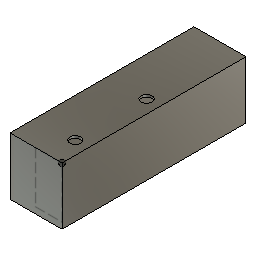
psu-box-115x31x37 (Autodesk Fusion 360 design; units mm, degrees)
Autodesk Fusion 360 part; units mm, degrees
sketch "Sketch1" plane through (0, 0, 0) normal (0, 0, 1) x (1, 0, 0)
  line L0 (0, 0) -> (33.5, 0)
  line L1 (33.5, 0) -> (33.5, 118.5)
  line L2 (33.5, 118.5) -> (0, 118.5)
  line L3 (0, 118.5) -> (0, 0)
  dimension "d1" = 33.5
  dimension "d2" = 118.5
  constraint horizontal L0
  constraint vertical L1
  constraint horizontal L2
  constraint vertical L3
  constraint coincident L0.start L3.end
  measures "d1" distance of L0.start L0.end
  measures "d2" distance of L0.start L2.end
extrude "Extrude2" add sketch "Sketch1" along normal blind 37
shell "Shell2" thickness 1.5 removed faces 1 at (11.1667, 79, 0)
sketch "Sketch2" plane through (0, 0, 37) normal (0, 0, 1) x (-1, 0, 0)
  line L0 (0, -118.5) -> (0, 0)
  line L1 (0, 0) -> (-33.5, 0)
  line L2 (-33.5, 0) -> (-33.5, -118.5)
  line L3 (-33.5, -118.5) -> (0, -118.5)
  line L4 (0, 0) -> (-25, 0) construction
  line L5 (-25, 0) -> (-25, -118.5) construction
  line L6 (-25, -118.5) -> (0, -118.5) construction
  line L7 (0, -118.5) -> (0, 0) construction
  line L8 (0, 0) -> (-25, 0) construction
  line L9 (-25, 0) -> (-25, -17) construction
  line L10 (-25, -17) -> (0, -17) construction
  line L11 (0, -17) -> (0, 0) construction
  line L12 (0, 0) -> (-25, 0) construction
  line L13 (-25, 0) -> (-25, -63) construction
  line L14 (-25, -63) -> (0, -63) construction
  line L15 (0, -63) -> (0, 0) construction
  circle A0 centre (-25, -63) radius 3.5
  circle A1 centre (-25, -17) radius 3.5
  dimension "d9" = 25
  dimension "d10" = 17
  dimension "d11" = 63
  dimension "d12" = 7
  dimension "d13" = 7
  constraint horizontal L4
  constraint vertical L5
  constraint horizontal L6
  constraint vertical L7
  constraint coincident L0.end L1.start
  constraint horizontal L8
  constraint vertical L9
  constraint horizontal L10
  constraint vertical L11
  constraint horizontal L12
  constraint vertical L13
  constraint horizontal L14
  constraint vertical L15
  constraint coincident L13.end L14.start
  constraint coincident L9.end L10.start
  measures "d9" distance of L0.end L4.end
  measures "d10" distance of L0.end L10.end
  measures "d11" distance of L0.end L14.end
  measures "d12" diameter of A0
  measures "d13" diameter of A1
extrude "Extrude3" cut sketch "Sketch2" against normal blind 10 contours A0 | A1
sketch "Sketch4" plane through (0, 1.5, 0) normal (0, 1, 0) x (-1, 0, 0)
  line L0 (-32, 0) -> (-1.5, 0)
  line L1 (-1.5, 0) -> (-1.5, 35.5)
  line L2 (-1.5, 35.5) -> (-32, 35.5)
  line L3 (-32, 35.5) -> (-32, 0)
  line L4 (-32, 35.5) -> (-15, 35.5) construction
  line L5 (-15, 35.5) -> (-15, 2.5) construction
  line L6 (-15, 2.5) -> (-32, 2.5) construction
  line L7 (-32, 2.5) -> (-32, 35.5) construction
  dimension "d16" = 17
  dimension "d17" = 33
  constraint horizontal L4
  constraint vertical L5
  constraint horizontal L6
  constraint vertical L7
  constraint coincident L2.end L3.start
  measures "d16" distance of L2.end L4.end
  measures "d17" distance of L2.end L6.end
